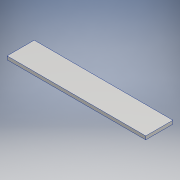
# Autodesk Inventor part: BK-BK120-Back
Saved by Autodesk Inventor 2017 (Build 210142000, 142)
## iProperties
Created: 2016-09-24
Part Number: BK-BK120-Back
Material: Aluminum 6061
Document SubType Name: Modeling
Designer: vslabsal
Density: 2.7 g/cm^3
Appearance: Aluminum - Flat
Author: vslabsal
Autodesk Inventor part; units mm, degrees
ref_plane "YZ Plane" through (0, 0, 0) normal (1, 0, 0) x (0, 1, 0)
ref_plane "XZ Plane" through (0, 0, 0) normal (0, 1, 0) x (-1, 0, 0)
ref_plane "XY Plane" through (0, 0, 0) normal (0, 0, 1) x (1, 0, 0)
sketch "Sketch1" plane through (0, 0, 0) normal (0, 0, 1) x (1, 0, 0)
  line L0 (-194.31, -38.1) -> (194.31, -38.1)
  line L1 (194.31, -38.1) -> (194.31, 38.1)
  line L2 (194.31, 38.1) -> (-194.31, 38.1)
  line L3 (-194.31, 38.1) -> (-194.31, -38.1)
  line L4 (-194.31, -38.1) -> (194.31, 38.1) construction
  line L5 (194.31, -38.1) -> (-194.31, 38.1) construction
  point P0 (0, 0)
  dimension "d0" = 388.62
  dimension "d1" = 76.2
  constraints: 12 end point, 2 midpoint, 2 parallel, 1 horizontal, 1 perpendicular
  measures "d0" distance of L0.start L0.end
  measures "d1" distance of L0.end L1.end
extrude "Extrusion2" add sketch "Sketch1" along normal blind 9.525
body "Solid2"
